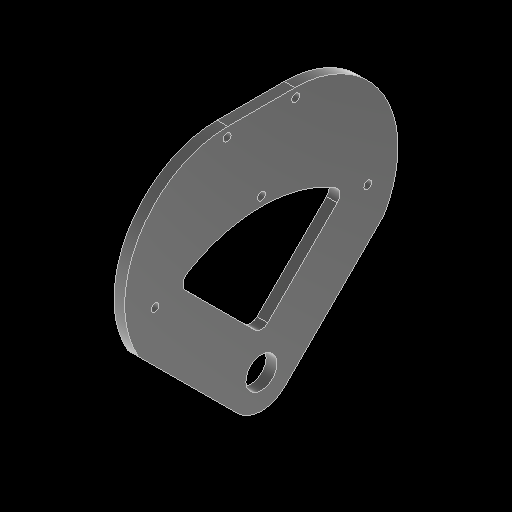
# Autodesk Inventor part: UHMWBearingUpright
Saved by Autodesk Inventor 2022 (Build 260153000, 153)
## iProperties
Created: 2021-02-15
Part Number: UHMWBearingUpright
Material: UHMW, Black
Document SubType Name: Modeling
Designer: Esketitttttt
Density: 0.94 g/cm^3
Appearance: Smooth - Black
Mass: 18.4109 g
Surface Area: 122.376 cm^2
Volume: 19.586 cm^3
Author: Esketitttttt
Autodesk Inventor part; units mm, degrees
ref_plane "YZ Plane" through (0, 0, 0) normal (1, 0, 0) x (0, 1, 0)
ref_plane "XZ Plane" through (0, 0, 0) normal (0, 1, 0) x (-1, 0, 0)
sketch "Sketch1" plane through (0, 0, 0) normal (1, 0, 0) x (0, 1, 0)
  circle A0 centre (0, 0) radius 5.5
  circle A1 centre (0, 0) radius 11.85
  line L0 (0, 0) -> (-81.28, 0) construction
  line L1 (0, -11.85) -> (-81.28, -11.85) construction
  line L2 (-81.28, -11.85) -> (-81.28, 11.85) construction
  line L3 (-81.28, 11.85) -> (0, 11.85) construction
  circle A2 centre (0, 0) radius 50.8 construction
  circle A3 centre (0, 0) radius 57.15 construction
  line L4 (-26.465, 43.3618) -> (-26.465, -43.3618) construction
  line L5 (-81.28, 11.85) -> (-81.28, -11.85)
  line L6 (-26.465, 43.3618) -> (8.3958, 8.3626)
  line L7 (8.3958, -8.3626) -> (-26.465, -43.3618)
  arc A4 (-26.465, 43.3618) -> (-81.28, 11.85) centre (-44.8148, 11.85) ccw
  arc A5 (-81.28, -11.85) -> (-26.465, -43.3618) centre (-44.8148, -11.85) ccw
  line L8 (-11.85, 0) -> (-41.3053, -29.5722)
  line L9 (-11.85, 0) -> (-41.3053, 29.5722)
  arc A6 (-41.3053, 29.5722) -> (-41.3053, -29.5722) centre (0, 0) ccw
  point P0 (-45.3426, -22.9062)
  dimension "d1" = 11
  dimension "d9" = 23.7
  dimension "d71" = 81.28
  dimension "d72" = 101.6
  dimension "d73" = 6.35
  dimension "d74" = 86.7236
  constraints: 20 end point, 15 point on circle, 7 centre point, 7 tangent, 4 midpoint, 3 coincident, 3 horizontal, 2 parallel, 2 vertical, 1 concentric, 1 perpendicular, 1 point on line
  measures "d1" diameter of A0
  measures "d9" diameter of A1
  measures "d71" distance of L0.start L0.end
  measures "d72" diameter of A2
  measures "d73" radial gap between concentric circles of A2 A3
  measures "d74" distance of L4.end L4.start
extrude "Extrusion1" add sketch "Sketch1" along normal blind 3.81
sketch "Sketch8" plane through (0, 0, 0) normal (-1, 0, 0) x (0, 0, 1)
  circle A0 centre (0, 0) radius 5.5 projected
  circle A1 centre (0, 0) radius 5.5 projected
  circle A2 centre (0, 0) radius 6.5
  dimension "d61" = 13
  constraints: 1 centre point, 1 coincident
  measures "d61" diameter of A2
extrude "BearingIndent" [suppressed]
fillet "Fillet3" radius 3.175 3 edges at (1.905, -41.3053, -29.5722) (1.905, -11.85, 0) (1.905, -41.3053, 29.5722)
ref_plane "Work Plane1" through (0, -53.8725, -73.7041) normal (1, 0, 0) x (0, 1, 0)
sketch "Sketch10" plane through (0, -53.8725, -73.7041) normal (1, 0, 0) x (0, 1, 0)
  circle A0 centre (-24.2325, 85.8211) radius 1.397 projected
  circle A1 centre (-24.2325, 61.587) radius 1.397 projected
  circle A2 centre (-0.1025, 73.7041) radius 1.397 projected
  circle A3 centre (15.1906, 111.3473) radius 1.397 projected
  circle A4 centre (15.1906, 36.0608) radius 1.397 projected
  point P0 (53.8725, 73.7041)
extrude "Extrusion7" cut sketch "Sketch10" along normal through all
sketch "Sketch9" plane through (0, 0, 0) normal (-1, 0, 0) x (0, 0, 1)
  line L0 (57.5605, -25.4) -> (15.4956, -67.9498) projected
  arc A0 (-2.8923, -53.1995) -> (15.4956, -67.9498) centre (0, 0) ccw projected
  arc A1 (-2.8923, -53.1995) -> (12.7651, 0) centre (-85.4426, 0) ccw projected
  arc A2 (-2.8923, -53.1995) -> (15.4956, -67.9498) centre (0, 0) ccw projected
  arc A3 (-2.8923, -53.1995) -> (12.7651, 0) centre (-85.4426, 0) ccw projected
  arc A4 (-38.0349, -86.0073) -> (12.7651, 0) centre (-85.4426, 0) ccw
  line L1 (57.5605, -25.4) -> (15.4956, -67.9498) projected
  arc A5 (-34.5747, -97.9062) -> (15.4956, -67.9498) centre (-38.5267, -34.4779) ccw
  arc A6 (-38.0349, -86.0073) -> (-34.5747, -97.9062) centre (-34.9696, -91.5685) ccw
  arc A7 (-34.9696, -91.5685) -> (2.1519, -74.6929) centre (-38.5267, -34.4779) ccw
  arc A8 (-34.9696, -91.5685) -> (19.1151, 0) centre (-85.4426, 0) ccw
  point P0 (3.0538, -70.7679)
  point P1 (-3.5107, -64.9575)
  point P2 (-2.8923, -53.1995)
  dimension "d64" = 50.8
  dimension "d66" = 6.35
  dimension "d67" = 6.35
  constraints: 10 point on circle, 5 centre point, 2 concentric, 2 tangent, 4 other
  measures "d64" horizontal distance of A1.end A4.start
  measures "d66" radius of A6
  measures "d67" radial gap between concentric circles of A5 A7
body "Solid1"
